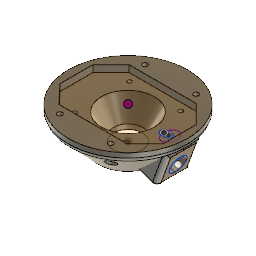
Unterteil (Autodesk Fusion 360 design; units mm, degrees)
Autodesk Fusion 360 part; units mm, degrees
sketch "Skizze1" plane through (0, 0, 0) normal (0, 0, 1) x (1, 0, 0)
  circle A0 centre (0, 0) radius 35
  dimension "d1" = 70
  measures "d1" diameter of A0
extrude "Extrusion1" add sketch "Skizze1" against normal blind 4 contours A0 picked at (8.845069, -11.842456) makes body 1
sketch "Skizze2" plane through (0, 0, 0) normal (0, 0, 1) x (-1, 0, 0)
  circle A0 centre (0, 0) radius 35
  line L0 (30.3, -9.7) -> (19.7, -20.3)
  line L1 (19.7, -20.3) -> (-19.7, -20.3)
  line L2 (-19.7, -20.3) -> (-30.5, -9.5)
  line L3 (-30.5, -9.5) -> (-30.5, 10)
  line L4 (-30.5, 10) -> (-20, 20.5)
  line L5 (-20, 20.5) -> (20.000001, 20.5)
  line L6 (20.000001, 20.5) -> (30.3, 9.685)
  line L7 (30.3, 9.685) -> (30.3, -9.7)
  line L8 (-34.150985, 4.873273) -> (34.150985, 4.873273)
  line L9 (-7.5, 4.370651) -> (-7.5, -12.129349)
  line L10 (-7.5, -12.129349) -> (7.5, -12.129349)
  line L11 (7.5, -12.129349) -> (7.5, 4.370651)
  line L12 (7.5, 4.370651) -> (-7.5, 4.370651)
  line L13 (20.000001, 20.5) -> (-20, 20.5)
  line L14 (-20, 20.5) -> (-30.5, 10)
  line L15 (-30.5, 10) -> (-30.5, -9.5)
  line L16 (-30.5, -9.5) -> (-19.7, -20.3)
  line L17 (-19.7, -20.3) -> (19.7, -20.3)
  line L18 (19.7, -20.3) -> (30.3, -9.7)
  line L19 (30.3, -9.7) -> (30.3, 9.685)
  line L20 (30.3, 9.685) -> (20.000001, 20.5)
  circle A1 centre (0, 0) radius 17.5
  circle A2 centre (0, 0) radius 15.5
  circle A3 centre (0, 0) radius 15.5
  circle A4 centre (0, 0) radius 8.5
  circle A5 centre (0, 0) radius 8.5
  line L21 (20.000001, 20.5) -> (-20, 20.5)
  line L22 (-20, 20.5) -> (-30.5, 10)
  line L23 (-30.5, 10) -> (-30.5, -9.5)
  line L24 (-30.5, -9.5) -> (-19.7, -20.3)
  line L25 (-19.7, -20.3) -> (19.7, -20.3)
  line L26 (19.7, -20.3) -> (30.3, -9.7)
  line L27 (30.3, -9.7) -> (30.3, 9.685)
  line L28 (30.3, 9.685) -> (20.000001, 20.5)
  line L29 (20.000001, 20.5) -> (-20, 20.5)
  line L30 (-20, 20.5) -> (-30.5, 10)
  line L31 (-30.5, 10) -> (-30.5, -9.5)
  line L32 (-30.5, -9.5) -> (-19.7, -20.3)
  line L33 (-19.7, -20.3) -> (19.7, -20.3)
  line L34 (19.7, -20.3) -> (30.3, -9.7)
  line L35 (30.3, -9.7) -> (30.3, 9.685)
  line L36 (30.3, 9.685) -> (20.000001, 20.5)
  circle A6 centre (15.197461, 15.999288) radius 1.25
  circle A7 centre (14.983329, -15.999996) radius 1.25
  circle A8 centre (-15, 16) radius 1.25
  circle A9 centre (-15.016671, -15.996902) radius 1.25
  circle A10 centre (0, 0) radius 15.5
  spline S0 degree 3 poles (-23.944611, -4.940796) (-23.534017, -4.856073) (-23.111966, -4.667346) (-22.369174, -4.07452) (-22.048213, -3.669751) (-21.578355, -2.798561) (-21.388315, -2.280541) (-21.140899, -1.161583) (-21.082473, -0.560713) (-21.082473, 0.560713) (-21.140899, 1.161583) (-21.388315, 2.280541) (-21.578355, 2.798561) (-22.048213, 3.669751) (-22.369174, 4.07452) (-23.111966, 4.667346) (-23.534017, 4.856073) (-24.463673, 5.047901) (-25.048289, 5.008337) (-26.185531, 4.611107) (-26.737395, 4.253676) (-27.626809, 3.36538) (-28.027748, 2.788446) (-28.577323, 1.46553) (-28.724455, 0.718892) (-28.724455, -0.718892) (-28.577323, -1.46553) (-28.027748, -2.788446) (-27.626809, -3.36538) (-26.737395, -4.253676) (-26.185531, -4.611107) (-25.048289, -5.008337) (-24.463673, -5.047901) (-23.944611, -4.940796) knots 0 0 0 0 0.18042905 0.18042905 0.36085809 0.36085809 0.52907196 0.52907196 0.69728582 0.69728582 0.86549968 0.86549968 1.03371355 1.03371355 1.21414259 1.21414259 1.39457164 1.39457164 1.62266519 1.62266519 1.85075873 1.85075873 2.06642627 2.06642627 2.28209381 2.28209381 2.49776135 2.49776135 2.71342888 2.71342888 2.94152243 2.94152243 3.16961598 3.16961598 3.16961598 3.16961598
  line L37 (-20, 20.5) -> (20.000001, 20.5)
  line L38 (20.000001, 20.5) -> (30.3, 9.685)
  line L39 (30.3, 9.685) -> (30.3, -9.7)
  line L40 (30.3, -9.7) -> (19.7, -20.3)
  line L41 (19.7, -20.3) -> (-19.7, -20.3)
  line L42 (-19.7, -20.3) -> (-30.5, -9.5)
  line L43 (-30.5, -9.5) -> (-30.5, 10)
  line L44 (-30.5, 10) -> (-20, 20.5)
  circle A11 centre (0, 0) radius 35
  circle A12 centre (0, 0) radius 15.5
  circle A13 centre (0, 0) radius 17.5
  circle A14 centre (-15, -25) radius 1.5
  circle A15 centre (-15, 25) radius 1.5
  circle A16 centre (15, -25) radius 1.5
  circle A17 centre (15, 25) radius 1.5
  line L45 (-20, 20.5) -> (20.000001, 20.5)
  line L46 (20.000001, 20.5) -> (30.3, 9.685)
  line L47 (30.3, 9.685) -> (30.3, -9.7)
  line L48 (30.3, -9.7) -> (19.7, -20.3)
  line L49 (19.7, -20.3) -> (-19.7, -20.3)
  line L50 (-19.7, -20.3) -> (-30.5, -9.5)
  line L51 (-30.5, -9.5) -> (-30.5, 10)
  line L52 (-30.5, 10) -> (-20, 20.5)
  circle A18 centre (0, 0) radius 35
extrude "Extrusion2" cut sketch "Skizze2" against normal blind 4 contours L0 L1 L2 L3 L7 L8 L15 L16 L17 L18 L19 A1 L23 L24 L25 L26 L27 L31 L32 L33 L34 L35 S0 L39 L40 L41 L42 L43 A13 L47 L48 L49 L50 L51 | L3 L4 L5 L6 L7 L8 L13 L14 L15 L19 L20 A1 L21 L22 L23 L27 L28 L29 L30 L31 L35 L36 S0 L37 L38 L39 L43 L44 A13 L45 L46 L47 L51 L52 | L8 A1 A2 A3 A10 A12 A13 | L8 A1 A2 A3 A10 A12 A13 | L8 L9 L10 L11 L12 A2 A3 A4 A5 A10 A12 | L8 A2 A3 A4 A5 A10 A12 | L8 L12 A4 A5 | L8 A4 A5 | L8 S0 | L8 S0 | L9 L11 L12 A4 A5 | L11 L12 A4 A5 | L9 L12 A4 A5 | L11 A4 A5 | L9 A4 A5 | L9 L10 L11 A4 A5 | A6 | A7 | A8 | A9 picked at (25.968821, -2.47406) picked at (20.823564, 10.733939) picked at (-11.286842, -12.445155) picked at (1.212201, 16.759662) picked at (8.880479, -8.787656) picked at (11.157313, 6.927985) picked at (-2.286527, 4.594884) picked at (-1.907798, 7.214086) picked at (-23.618103, 0.60012) picked at (-24.735228, 4.897274) picked at (-2.569924, 1.456884) picked at (7.384146, 4.329859) picked at (-7.384146, 4.329859) picked at (7.64418, 1.017885) picked at (-7.661586, -0.971463) picked at (0.203982, -10.912214) picked at (15.58299, 15.583786) picked at (15.340221, -15.942026) picked at (-15.375403, 16.180785) picked at (-14.618516, -16.235657) bodies 1
ref_plane "Arbeitsebene1" through (0, 0, -22) normal (0, 0, 1) x (1, 0, 0)
sketch "Skizze3" plane through (0, 0, -22) normal (0, 0, 1) x (1, 0, 0)
  circle A0 centre (0, 0) radius 17.5
  dimension "d9" = 35
  measures "d9" diameter of A0
loft "Erhebung1" add profiles "Skizze3" section 1 face at (-0.871851, 25.167378, -4) section 2 contours A0 picked at (4.422535, -5.921228) on bodies 1 bodies 1
fillet "Abrundung1" radius 3 1 edges at (-32.631457, 12.65654, -4) on bodies 1
sketch "Skizze4" plane through (0, 0, 0) normal (0, 1, 0) x (1, 0, 0)
  line L0 (32.593982, 7.21209) -> (26.0956, 25.066249)
  line L1 (32.593982, 7.21209) -> (57.000001, 7.21209) construction
  line L2 (26.0956, 25.066249) -> (14.91513, 20.996891)
  line L3 (-34.150985, 4.873273) -> (34.150985, 4.873273)
  line L4 (14.91513, 20.996891) -> (20.783647, 4.873273)
  line L5 (20.783647, 4.873273) -> (32.593982, 4.873273)
  line L6 (32.593982, 4.873273) -> (32.593982, 7.21209)
  dimension "d11" = 110
  dimension "d12" = 19
  measures "d11" angle of L0 L1
  measures "d12" distance of origin
extrude "Extrusion3" add sketch "Skizze4" along normal mid plane 20 separate body contours L0 L2 L3 L4 L5 L6 picked at (26.491076, 12.383871) makes body 2
fillet "Abrundung2" radius 2 2 edges at (20.505365, 10, -23.03157) (20.505365, -10, -23.03157) on bodies 2
fillet "Abrundung3" radius 2.5 5 edges at (29.686811, 10, -15.199477) (26.295951, 9.414214, -24.51579) (26.0956, 0, -25.066249) (26.295951, -9.414214, -24.51579) (29.686811, -10, -15.199477) on bodies 2
fillet "Abrundung4" radius 0.5 2 edges at (31.756528, -9.827273, -4.873273) (25.784222, -10, -4.873273) on bodies 2
sketch "Skizze5" plane through (31.099132, 0, -11.319158) normal (0.939693, 0, -0.34202) x (0, 1, 0)
  line L0 (-7.5, 4.370651) -> (-7.5, -12.129349)
  line L1 (-7.5, -12.129349) -> (7.5, -12.129349)
  line L2 (7.5, -12.129349) -> (7.5, 4.370651)
  line L3 (7.5, 4.370651) -> (-7.5, 4.370651)
  circle A0 centre (0, -5) radius 5
  dimension "d18" = 10
  measures "d18" diameter of A0
extrude "Extrusion4" cut sketch "Skizze5" against normal blind 17 contours A0 picked at (0.215557, -7.876405) bodies 1 2
sketch "Skizze6" plane through (0, 0, -4) normal (0, 0, 1) x (-1, 0, 0)
  line L0 (20.000001, 20.5) -> (-20, 20.5)
  line L1 (-20, 20.5) -> (-30.5, 10)
  line L2 (-30.5, 10) -> (-30.5, -9.5)
  line L3 (-30.5, -9.5) -> (-19.7, -20.3)
  line L4 (-19.7, -20.3) -> (19.7, -20.3)
  line L5 (19.7, -20.3) -> (30.3, -9.7)
  line L6 (30.3, -9.7) -> (30.3, 9.685)
  line L7 (30.3, 9.685) -> (20.000001, 20.5)
  circle A0 centre (0, 0) radius 15
  dimension "d21" = 30
  measures "d21" diameter of A0
sketch "Skizze7" plane through (0, 0, -22) normal (0, 0, -1) x (1, 0, 0)
  circle A0 centre (0, 0) radius 17.5
  circle A1 centre (0, 0) radius 15.5
  dimension "d22" = 31
  measures "d22" diameter of A1
extrude "Extrusion5" cut sketch "Skizze7" against normal blind 3 contours A1 picked at (0.668226, 1.387585) bodies 1 2
sketch "Skizze8" plane through (0, 0, -19) normal (0, 0, -1) x (1, 0, 0)
  circle A0 centre (0, 0) radius 15.5
  circle A1 centre (0, 0) radius 8.5
  dimension "d25" = 17
  measures "d25" diameter of A1
extrude "Extrusion8" cut sketch "Skizze8" against normal blind 2 contours A1 picked at (2.707456, 1.623535) bodies 1
extrude "Extrusion6" cut sketch "Skizze5" against normal blind 20 contours A0 picked at (0.215557, -7.876405) bodies 1
sketch "Skizze9" plane through (0, 0, 0) normal (0, 0, 1) x (1, 0, 0)
sketch "Skizze10" plane through (0, 0, 0) normal (0, 1, 0) x (1, 0, 0)
sketch "Skizze11" plane through (0, 0, -19) normal (0, 0, -1) x (1, 0, 0)
  circle A0 centre (0, 0) radius 15.5
  circle A1 centre (12.999995, -0.010948) radius 1.25
  circle A2 centre (-6.490517, 11.2638) radius 1.25
  circle A3 centre (-6.509479, -11.252852) radius 1.25
  circle A4 centre (0, 0) radius 8.5
  dimension "d30" = 2.5
  dimension "d32" = 360
  measures "d30" diameter of A1
extrude "Extrusion7" cut sketch "Skizze11" against normal blind 8 contours A1 | A2 | A3 picked at (12.585764, 0.326389) picked at (-6.078504, 11.080272) picked at (-6.889536, -11.495738) bodies 1
ref_plane "Arbeitsebene2" through (0, 0, -17) normal (0, 0, -1) x (1, 0, 0)
sketch "Skizze13" plane through (0, 0, 0) normal (0, 0, 1) x (1, 0, 0)
extrude "Extrusion9" cut sketch "Skizze8" against normal blind 42 contours A1 picked at (2.707456, 1.623535) bodies 1
sketch "Skizze14" plane through (0, 0, -4) normal (0, 0, 1) x (-1, 0, 0)
  circle A0 centre (0, 0) radius 8.5
  line L0 (20.000001, 20.5) -> (-20, 20.5)
  line L1 (-20, 20.5) -> (-30.5, 10)
  line L2 (-30.5, 10) -> (-30.5, -9.5)
  line L3 (-30.5, -9.5) -> (-19.7, -20.3)
  line L4 (-19.7, -20.3) -> (19.7, -20.3)
  line L5 (19.7, -20.3) -> (30.3, -9.7)
  line L6 (30.3, -9.7) -> (30.3, 9.685)
  line L7 (30.3, 9.685) -> (20.000001, 20.5)
  circle A1 centre (0, 0) radius 15
  circle A2 centre (14.983329, -15.999996) radius 1.25
  circle A3 centre (-15.016671, -15.996902) radius 1.25
  circle A4 centre (-15, 16) radius 1.25
  circle A5 centre (15.197461, 15.999288) radius 1.25
  dimension "d43" = 30
  dimension "d46" = 30
  dimension "d47" = 32
  dimension "d48" = 2.5
  dimension "d49" = 2.5
  dimension "d50" = 2.5
  dimension "d51" = 2.5
  measures "d43" diameter of A1
  measures "d48" diameter of A2
  measures "d49" diameter of A3
  measures "d50" diameter of A4
  measures "d51" diameter of A5
extrude "Extrusion10" cut sketch "Skizze14" against normal blind 10 contours A2 | A3 | A4 | A5 picked at (15.340221, -15.942026) picked at (-14.618516, -16.235657) picked at (-15.375403, 16.180785) picked at (15.58299, 15.583786) bodies 1
chamfer "Fase1" distance 7 angle 60 1 edges at (-7.924782, 3.073731, -4) measured on face at (23.166667, -0.166667, -4) on bodies 1
sketch "Skizze15" plane through (0, 0, -4) normal (0, 0, 1) x (-1, 0, 0)
  line L0 (20.000001, 20.5) -> (-20, 20.5)
  line L1 (-20, 20.5) -> (-30.5, 10)
  line L2 (-30.5, 10) -> (-30.5, -9.5)
  line L3 (-30.5, -9.5) -> (-19.7, -20.3)
  line L4 (-19.7, -20.3) -> (19.7, -20.3)
  line L5 (19.7, -20.3) -> (30.3, -9.7)
  line L6 (30.3, -9.7) -> (30.3, 9.685)
  line L7 (30.3, 9.685) -> (20.000001, 20.5)
  circle A0 centre (15.197461, 15.999288) radius 1.25
  circle A1 centre (14.983329, -15.999996) radius 1.25
  circle A2 centre (-15, 16) radius 1.25
  circle A3 centre (-15.016671, -15.996902) radius 1.25
  circle A4 centre (0, 0) radius 15.5
  line L8 (-23.828841, -2) -> (-21.082473, -2)
  arc A5 (-21.082473, -2) -> (-21.082473, 2) centre (-21.082473, 0) ccw
  line L9 (-21.082473, 2) -> (-23.828841, 2)
  arc A6 (-23.828841, 2) -> (-23.828841, -2) centre (-23.828841, 0) ccw
  line L10 (-23.828841, 0) -> (-21.082473, 0) construction
  spline S0 degree 3 poles (-23.944611, -4.940796) (-23.534017, -4.856073) (-23.111966, -4.667346) (-22.369174, -4.07452) (-22.048213, -3.669751) (-21.578355, -2.798561) (-21.388315, -2.280541) (-21.140899, -1.161583) (-21.082473, -0.560713) (-21.082473, 0.560713) (-21.140899, 1.161583) (-21.388315, 2.280541) (-21.578355, 2.798561) (-22.048213, 3.669751) (-22.369174, 4.07452) (-23.111966, 4.667346) (-23.534017, 4.856073) (-24.463673, 5.047901) (-25.048289, 5.008337) (-26.185531, 4.611107) (-26.737395, 4.253676) (-27.626809, 3.36538) (-28.027748, 2.788446) (-28.577323, 1.46553) (-28.724455, 0.718892) (-28.724455, -0.718892) (-28.577323, -1.46553) (-28.027748, -2.788446) (-27.626809, -3.36538) (-26.737395, -4.253676) (-26.185531, -4.611107) (-25.048289, -5.008337) (-24.463673, -5.047901) (-23.944611, -4.940796) knots 0 0 0 0 0.18042905 0.18042905 0.36085809 0.36085809 0.52907196 0.52907196 0.69728582 0.69728582 0.86549968 0.86549968 1.03371355 1.03371355 1.21414259 1.21414259 1.39457164 1.39457164 1.62266519 1.62266519 1.85075873 1.85075873 2.06642627 2.06642627 2.28209381 2.28209381 2.49776135 2.49776135 2.71342888 2.71342888 2.94152243 2.94152243 3.16961598 3.16961598 3.16961598 3.16961598
extrude "Extrusion11" cut sketch "Skizze15" against normal blind 5 contours L8 L9 A6 S0 | L8 A5 L9 S0 picked at (-22.913897, 0.052742) picked at (-20.522869, -0.589348) bodies 1 2
sketch "Skizze16" plane through (0, 0, 0) normal (0, 0, 1) x (-1, 0, 0)
  line L0 (-20, 20.5) -> (20.000001, 20.5)
  line L1 (20.000001, 20.5) -> (30.3, 9.685)
  line L2 (30.3, 9.685) -> (30.3, -9.7)
  line L3 (30.3, -9.7) -> (19.7, -20.3)
  line L4 (19.7, -20.3) -> (-19.7, -20.3)
  line L5 (-19.7, -20.3) -> (-30.5, -9.5)
  line L6 (-30.5, -9.5) -> (-30.5, 10)
  line L7 (-30.5, 10) -> (-20, 20.5)
  circle A0 centre (0, 0) radius 35
  circle A1 centre (15, -25) radius 1.5
  circle A2 centre (-15, -25) radius 1.5
  circle A3 centre (15, 25) radius 1.5
  circle A4 centre (-15, 25) radius 1.5
  dimension "d56" = 30
  dimension "d57" = 50
  dimension "d58" = 3
  dimension "d59" = 3
  dimension "d60" = 3
  dimension "d61" = 3
  measures "d58" diameter of A1
  measures "d59" diameter of A2
  measures "d60" diameter of A3
  measures "d61" diameter of A4
extrude "Extrusion12" cut sketch "Skizze16" against normal blind 28 contours A1 | A2 | A3 | A4 picked at (15.383155, -25.561985) picked at (-14.505584, -25.074522) picked at (15.383155, 24.438015) picked at (-14.505584, 24.925478) bodies 1
sketch "Skizze17" plane through (0, 0, -22) normal (0, 0, -1) x (1, 0, 0)
  circle A0 centre (0, 0) radius 15.5
  circle A1 centre (0, 0) radius 17.5
  circle A2 centre (-15, 25) radius 2.9
  circle A3 centre (15, 25) radius 2.9
  circle A4 centre (-15, -25) radius 2.9
  circle A5 centre (15, -25) radius 2.9
  dimension "d64" = 5.8
  dimension "d65" = 5.8
  dimension "d66" = 5.8
  dimension "d67" = 5.8
  measures "d64" diameter of A2
  measures "d65" diameter of A3
  measures "d66" diameter of A4
  measures "d67" diameter of A5
extrude "Extrusion13" cut sketch "Skizze17" against normal blind 18 contours A2 | A3 | A4 | A5 picked at (-14.087077, 25.140856) picked at (15.923721, 24.71507) picked at (-14.20645, -23.779005) picked at (15.923721, -25.28493) bodies 1
sketch "Skizze18" plane through (0, 0, 0) normal (0, 0, 1) x (-1, 0, 0)
  circle A0 centre (-15, -25) radius 1.5
  circle A1 centre (-15, 25) radius 1.5
  circle A2 centre (15, -25) radius 1.5
  circle A3 centre (15, 25) radius 1.5
  line L0 (-20, 20.5) -> (20.000001, 20.5)
  line L1 (20.000001, 20.5) -> (30.3, 9.685)
  line L2 (30.3, 9.685) -> (30.3, -9.7)
  line L3 (30.3, -9.7) -> (19.7, -20.3)
  line L4 (19.7, -20.3) -> (-19.7, -20.3)
  line L5 (-19.7, -20.3) -> (-30.5, -9.5)
  line L6 (-30.5, -9.5) -> (-30.5, 10)
  line L7 (-30.5, 10) -> (-20, 20.5)
  circle A4 centre (0, 0) radius 35
